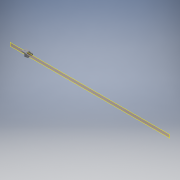
# Autodesk Inventor part: YIdler
Saved by Autodesk Inventor 2016 (Build 200138000, 138)
## iProperties
Created: 2016-05-31
Part Number: YIdler
Material: Generic
Document SubType Name: Modeling
Designer: Scott
Density: 1 g/cm^3
Appearance: Default
Author: Scott
Autodesk Inventor part; units mm, degrees
ref_plane "YZ Plane" through (0, 0, 0) normal (1, 0, 0) x (0, 1, 0)
ref_plane "XZ Plane" through (0, 0, 0) normal (0, 1, 0) x (-1, 0, 0)
ref_plane "XY Plane" through (0, 0, 0) normal (0, 0, 1) x (1, 0, 0)
ref_plane "Work Plane1" through (0, 0, 0) normal (0, 0, 1) x (1, 0, 0)
sketch "Sketch1" plane through (0, 0, 0) normal (0, 0, 1) x (1, 0, 0)
  line L0 (-521.65, -0.245) -> (-521.65, -0.245) projected
  line L1 (-521.65, 19.755) -> (-521.65, -0.245) projected
  line L2 (-521.65, 19.755) -> (-521.65, 19.755) projected
  line L3 (-521.65, -0.245) -> (-521.65, 19.755) projected
  line L4 (-501.65, 19.755) -> (-501.65, 19.755) projected
  line L5 (-501.65, -0.245) -> (-501.65, 19.755) projected
  line L6 (-501.65, -0.245) -> (-501.65, -0.245) projected
  line L7 (-501.65, 19.755) -> (-501.65, -0.245) projected
  line L8 (-521.65, -0.245) -> (-521.65, -0.245) projected
  line L9 (-521.65, 19.755) -> (-521.65, -0.245) projected
  line L10 (-521.65, 19.755) -> (-521.65, 19.755) projected
  line L11 (-521.65, -0.245) -> (-521.65, 19.755) projected
  line L12 (-501.65, 19.755) -> (-499.11, 19.755)
  line L13 (-499.11, 19.755) -> (-499.11, -0.245)
  line L14 (-499.11, -0.245) -> (-501.65, -0.245)
  line L15 (-501.65, -0.245) -> (-501.65, 19.755)
  line L16 (-499.11, 19.755) -> (-521.65, 19.755)
  line L17 (-521.65, 19.755) -> (-521.65, 24.835)
  line L18 (-521.65, 24.835) -> (-499.11, 24.835)
  line L19 (-499.11, 24.835) -> (-499.11, 19.755)
  point P0 (0, 0)
  dimension "d0" = 2.54
  dimension "d1" = 5.08
  constraints: 16 end point, 4 parallel, 2 horizontal, 2 perpendicular
  measures "d0" distance of L13.end L14.end
  measures "d1" distance of L16.end L17.end
extrude "Extrusion1" add sketch "Sketch1" along normal mid plane 30.48
sketch "Sketch2" plane through (-521.65, 24.835, 15.24) normal (0, 1, 0) x (1, 0, 0)
  line L0 (0, 30.48) -> (0, 0) projected
  line L1 (22.54, 0) -> (0, 0) projected
  line L2 (22.54, 30.48) -> (22.54, 0) projected
  line L3 (0, 30.48) -> (22.54, 30.48) projected
  line L4 (20, 345.44) -> (20, -314.96) projected
  line L5 (0, 30.48) -> (0, 0) projected
  line L6 (0, 15.24) -> (20, 15.24)
  circle A0 centre (10, 15.24) radius 2.5
  point P0 (521.65, 15.24)
  dimension "d4" = 5
  constraints: 3 midpoint, 2 end point, 1 centre point
  measures "d4" diameter of A0
extrude "Extrusion2" cut sketch "Sketch2" against normal blind 25.4 contours A0 L6 | L6 A0
sketch "Sketch3" plane through (-501.65, -0.245, 15.24) normal (-1, 0, 0) x (0, 0, 1)
  line L0 (-345.44, 0) -> (314.96, 0) projected
  line L1 (-30.48, 20) -> (0, 20) projected
  line L2 (-15.24, 20) -> (-15.24, 0)
  line L3 (-30.48, 0) -> (0, 0) projected
  circle A0 centre (-15.24, 10) radius 2.5
  point P0 (-15.24, 0.245)
  dimension "d7" = 5
  constraints: 3 midpoint, 2 end point, 1 centre point
  measures "d7" diameter of A0
extrude "Extrusion3" cut sketch "Sketch3" against normal blind 25.4
sketch "Sketch4" plane through (0, 0, -15.24) normal (0, 0, -1) x (-1, 0, 0)
  line L0 (499.11, -0.245) -> (499.11, 24.835) projected
  line L1 (499.11, 24.835) -> (499.11, -0.245) projected
  line L2 (499.11, 12.295) -> (480.06, 12.295)
  line L3 (499.11, 12.295) -> (518.16, 12.295) construction
  arc A0 (478.2847, 20.0955) -> (478.2847, 4.4944) centre (480.06, 12.295) ccw
  circle A1 centre (480.06, 12.295) radius 2.5
  line L4 (499.11, 24.835) -> (478.2847, 20.0955)
  line L5 (499.11, -0.245) -> (478.2847, 4.4944)
  point P0 (0, 0)
  dimension "d10" = 19.05
  dimension "d11" = 180
  dimension "d12" = 16
  dimension "d13" = 5
  constraints: 8 end point, 2 centre point, 2 coincident, 2 horizontal, 2 point on circle, 2 tangent, 1 collinear, 1 midpoint
  measures "d10" distance of L2.start L2.end
  measures "d11" angle of L2 L3
  measures "d12" diameter of A0
  measures "d13" diameter of A1
extrude "Extrusion4" add sketch "Sketch4" against normal blind 5.08
sketch "Sketch5" plane through (0, 0, 15.24) normal (0, 0, 1) x (1, 0, 0)
  circle A0 centre (-480.06, 12.295) radius 2.5 projected
  line L0 (-499.11, -0.245) -> (-499.11, 24.835) projected
  line L1 (-499.11, -0.245) -> (-478.2847, 4.4944) projected
  arc A1 (-478.2847, 4.4944) -> (-478.2847, 20.0955) centre (-480.06, 12.295) ccw projected
  line L2 (-478.2847, 20.0955) -> (-499.11, 24.835) projected
  point P0 (0, 0)
extrude "Extrusion5" add sketch "Sketch5" against normal blind 5.08
sketch "Sketch6" plane through (-499.11, -0.245, 10.16) normal (0.2219, -0.9751, 0) x (0.9751, 0.2219, 0)
  line L0 (0, 5.08) -> (21.3578, 5.08) projected
  line L1 (0, 0) -> (0, 5.08) projected
  line L2 (21.3578, 0) -> (0, 0) projected
  line L3 (21.3578, 5.08) -> (21.3578, 0) projected
  line L4 (21.3578, -25.4) -> (0, -25.4) projected
  line L5 (21.3578, -25.4) -> (21.3578, -20.32) projected
  line L6 (0, -20.32) -> (21.3578, -20.32) projected
  line L7 (0, -25.4) -> (0, -20.32) projected
  line L8 (0, -20.32) -> (0, 0) projected
  line L9 (21.3578, -25.4) -> (0, -25.4) projected
  line L10 (0, 5.08) -> (5.08, 5.08)
  line L11 (5.08, 5.08) -> (5.08, -25.4)
  line L12 (5.08, -25.4) -> (0, -25.4)
  line L13 (0, -25.4) -> (0, 5.08)
  point P0 (486.7204, -10.16)
  dimension "d18" = 5.08
  constraints: 8 end point, 2 parallel, 1 horizontal, 1 perpendicular, 1 point on line
  measures "d18" distance of L11.end L12.end
extrude "Extrusion6" add sketch "Sketch6" against normal blind 2.54 contours L0 L11 L2 L1 | L2 L11 L6 L8 | L6 L11 L4 L7
sketch "Sketch7" plane through (-499.11, 24.835, -10.16) normal (0.2219, 0.9751, 0) x (0.9751, -0.2219, 0)
  line L0 (21.3578, -25.4) -> (0, -25.4) projected
  line L1 (21.3578, -25.4) -> (21.3578, -20.32) projected
  line L2 (0, -20.32) -> (21.3578, -20.32) projected
  line L3 (0, -20.32) -> (0, -25.4) projected
  line L4 (0, 5.08) -> (21.3578, 5.08) projected
  line L5 (0, 5.08) -> (0, 0) projected
  line L6 (21.3578, 0) -> (0, 0) projected
  line L7 (21.3578, 5.08) -> (21.3578, 0) projected
  line L8 (0, -25.4) -> (5.08, -25.4)
  line L9 (5.08, -25.4) -> (5.08, 5.08)
  line L10 (5.08, 5.08) -> (0, 5.08)
  line L11 (0, 5.08) -> (0, -25.4)
  point P0 (492.1771, -10.16)
  dimension "d21" = 5.08
  constraints: 8 end point, 2 parallel, 1 horizontal, 1 perpendicular, 1 point on line
  measures "d21" distance of L10.end L9.end
extrude "Extrusion7" add sketch "Sketch7" against normal blind 2.54 contours L0 L3 L2 L9 | L2 L11 L6 L9 | L6 L5 L4 L9
body "Solid1"
